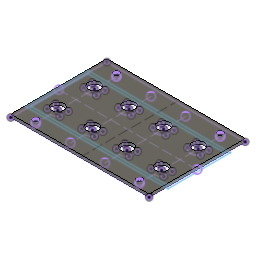
Compact ABR enclosure (Autodesk Fusion 360 archive; units mm, degrees)
design "ABR box faceplate"
Autodesk Fusion 360 part; units mm, degrees
sketch "Sketch1" plane through (0, 0, 0) normal (0, 0, 1) x (1, 0, 0)
  circle A0 centre (9, 34.525) radius 3.95
  circle A1 centre (9, 15.475) radius 3.95
  line L0 (9, 34.525) -> (9, 15.475) construction
  circle A2 centre (9, 45.975) radius 1.5
  circle A3 centre (9, 4.025) radius 1.5
  line L1 (-1.2896, 25) -> (19.2896, 25) construction
  line L2 (9, 45.975) -> (9, 4.025) construction
  line L3 (5.7, 40.3994) -> (5.7, 10.52)
  line L4 (5.7, 10.52) -> (12.3, 10.52) construction
  line L5 (12.3, 10.52) -> (12.3, 40.3994)
  line L6 (12.3, 40.3994) -> (5.7, 40.3994) construction
  line L7 (5.05, 34.525) -> (12.95, 34.525) construction
  circle A4 centre (27, 34.525) radius 3.95
  line L8 (23.7, 40.3994) -> (23.7, 10.52)
  line L9 (30.3, 10.52) -> (30.3, 40.3994)
  circle A5 centre (27, 15.475) radius 3.95
  circle A6 centre (27, 4.025) radius 1.5
  circle A7 centre (27, 45.975) radius 1.5
  circle A8 centre (45, 34.525) radius 3.95
  line L10 (41.7, 40.3994) -> (41.7, 10.52)
  line L11 (48.3, 10.52) -> (48.3, 40.3994)
  circle A9 centre (45, 15.475) radius 3.95
  circle A10 centre (45, 4.025) radius 1.5
  circle A11 centre (45, 45.975) radius 1.5
  line L12 (0, 50) -> (72, 50)
  line L13 (72, 50) -> (72, 0)
  line L14 (72, 0) -> (0, 0)
  line L15 (0, 0) -> (0, 50)
  line L16 (27, 45.975) -> (27, 4.025) construction
  line L17 (45, 45.975) -> (45, 4.025) construction
  circle A12 centre (63, 34.525) radius 3.95
  line L18 (59.7, 40.3994) -> (59.7, 10.52)
  line L19 (66.3, 10.52) -> (66.3, 40.3994)
  circle A13 centre (63, 15.475) radius 3.95
  circle A14 centre (63, 4.025) radius 1.5
  circle A15 centre (63, 45.975) radius 1.5
  line L20 (63, 45.975) -> (63, 4.025) construction
  line L21 (36, 50) -> (36, 0) construction
  line L22 (0, 25) -> (72, 25) construction
  line L23 (9, 15.475) -> (27, 15.475) construction
  line L24 (18, 15.475) -> (18, 27.912) construction
  point P0 (9, 5.525)
  point P1 (9, 11.525)
  point P2 (27, 34.525)
  point P3 (27, 15.475)
  point P4 (45, 34.525)
  point P5 (45, 15.475)
  point P6 (63, 34.525)
  point P7 (63, 15.475)
  point P8 (45, -15.475)
  point P9 (0, -50)
  point P10 (0, -25)
  point P11 (45, -45.975)
  point P12 (45, -34.525)
  point P13 (0, 50)
  dimension "d4" = 7.9
  dimension "d5" = 7.9
  dimension "d6" = 19.05
  dimension "d7" = 6
  dimension "d8" = 3
  dimension "d9" = 0.65
  dimension "d12" = 18
  dimension "d13" = 0
  dimension "d19" = 50
  dimension "d24" = 41.95
  dimension "d34" = 9
  dimension "d35" = 9
  dimension "d36" = 9
  constraint coincident A0.centre L0.start
  constraint coincident A1.centre L0.end
  constraint vertical L0
  constraint coincident L0 A2.centre
  constraint coincident L0 A3.centre
  constraint horizontal L1
  constraint midpoint L0 L1
  constraint symmetric A2 A3 L1
  constraint coincident A2.centre L2.start
  constraint coincident A3.centre L2.end
  constraint coincident A3 P0
  constraint coincident L2 P0
  constraint coincident L2 P1
  constraint coincident A1 P1
  constraint vertical L3
  constraint perpendicular L3 L4
  constraint perpendicular L4 L5
  constraint symmetric L2 L3 L5
  constraint horizontal L6
  constraint coincident A0 L7.start
  constraint coincident A0 L7.end
  constraint perpendicular L5 L7
  constraint coincident A0.centre L7
  constraint horizontal L12
  constraint vertical L13
  constraint horizontal L14
  constraint vertical L15
  constraint midpoint L12 L21.start
  constraint midpoint L14 L21.end
  constraint midpoint L15 L22.start
  constraint midpoint L13 L22.end
  constraint coincident L1 L22.start
  constraint coincident P3 A5.centre
  constraint midpoint L23 L24.start
  constraint perpendicular L1 L24
  constraint coincident L14.end L15.start
  measures "d4" diameter of A0
  measures "d5" diameter of A1
  measures "d6" distance of A0.centre A1.centre
  measures "d7" distance of P0 P1
  measures "d8" diameter of A3
  measures "d9" distance of L5 L7.end
  measures "d19" distance of P13 L14.end
  measures "d24" distance of A2.centre A3.centre
  measures "d34" distance of L0 L24
  measures "d35" distance of L2 L15
  measures "d36" distance of L13 L20
extrude "Extrude1" add sketch "Sketch1" along normal blind 1.5 contours A0 L5 | A0 A1 L3 L5 | A0 L3 | A1 L5 | A1 L3 | A4 L9 | A4 L8 L9 A5 | A4 L8 | L9 A5 | L8 A5 | A6 | A7 | A8 L11 | A8 L10 L11 A9 | A8 L10 | L11 A9 | L10 A9 | A10 | A11 | L12 L13 L14 L15 | A12 L19 | A12 L18 L19 A13 | A12 L18 | L19 A13 | L18 A13 makes body 1
sketch "Sketch2" plane through (0, 0, 0) normal (0, 0, -1) x (1, 0, 0)
  circle A0 centre (9, -4.025) radius 1.5
  circle A1 centre (63, -4.025) radius 1.5
  arc A2 (12.3, -13.3042) -> (5.7, -13.3042) centre (9, -15.475) ccw construction
  line L0 (12.3, -13.3042) -> (12.3, -17.6458) construction
  arc A3 (5.7, -17.6458) -> (12.3, -17.6458) centre (9, -15.475) ccw construction
  line L1 (5.7, -17.6458) -> (5.7, -13.3042) construction
  line L2 (30.3, -13.3042) -> (30.3, -17.6458) construction
  arc A4 (23.7, -17.6458) -> (30.3, -17.6458) centre (27, -15.475) ccw construction
  line L3 (23.7, -17.6458) -> (23.7, -13.3042) construction
  arc A5 (30.3, -13.3042) -> (23.7, -13.3042) centre (27, -15.475) ccw construction
  circle A6 centre (63, -45.975) radius 1.5
  line L4 (48.3, -13.3042) -> (48.3, -17.6458) construction
  arc A7 (41.7, -17.6458) -> (48.3, -17.6458) centre (45, -15.475) ccw construction
  line L5 (41.7, -17.6458) -> (41.7, -13.3042) construction
  arc A8 (48.3, -13.3042) -> (41.7, -13.3042) centre (45, -15.475) ccw construction
  circle A9 centre (9, -45.975) radius 1.5
  line L6 (66.3, -13.3042) -> (66.3, -17.6458) construction
  arc A10 (59.7, -17.6458) -> (66.3, -17.6458) centre (63, -15.475) ccw construction
  line L7 (59.7, -17.6458) -> (59.7, -13.3042) construction
  arc A11 (66.3, -13.3042) -> (59.7, -13.3042) centre (63, -15.475) ccw construction
  line L8 (72, 0) -> (0, 0)
  line L9 (0, 0) -> (0, -50)
  line L10 (0, -50) -> (72, -50)
  line L11 (72, -50) -> (72, 0)
  line L12 (0.4311, -10.2537) -> (71.5689, -10.2537)
  line L13 (71.5689, -10.2537) -> (71.5689, -39.7463)
  line L14 (71.5689, -39.7463) -> (0.4311, -39.7463)
  line L15 (0.4311, -39.7463) -> (0.4311, -10.2537)
  line L16 (0, -25) -> (72, -25) construction
  line L17 (27, -45.975) -> (27, -4.025) construction
  line L18 (45, -45.975) -> (45, -4.025) construction
  line L19 (63, -45.975) -> (63, -4.025) construction
  line L20 (9, -45.975) -> (9, -4.025) construction
  line L21 (36, 0) -> (36, -50) construction
  line L22 (73.0689, -8.7537) -> (73.0689, -41.2463)
  line L23 (73.0689, -41.2463) -> (-1.0689, -41.2463)
  line L24 (-1.0689, -41.2463) -> (-1.0689, -8.7537)
  line L25 (-1.0689, -8.7537) -> (73.0689, -8.7537)
  arc A12 (12.3, -32.3542) -> (5.7, -32.3542) centre (9, -34.525) ccw
  line L26 (12.3, -32.3542) -> (12.3, -36.6958)
  arc A13 (5.7, -36.6958) -> (12.3, -36.6958) centre (9, -34.525) ccw
  line L27 (5.7, -36.6958) -> (5.7, -32.3542)
  arc A14 (66.3, -32.3542) -> (59.7, -32.3542) centre (63, -34.525) ccw
  line L28 (66.3, -32.3542) -> (66.3, -36.6958)
  arc A15 (59.7, -36.6958) -> (66.3, -36.6958) centre (63, -34.525) ccw
  line L29 (59.7, -36.6958) -> (59.7, -32.3542)
  arc A16 (30.3, -32.3542) -> (23.7, -32.3542) centre (27, -34.525) ccw
  line L30 (30.3, -32.3542) -> (30.3, -36.6958)
  arc A17 (23.7, -36.6958) -> (30.3, -36.6958) centre (27, -34.525) ccw
  line L31 (23.7, -36.6958) -> (23.7, -32.3542)
  arc A18 (48.3, -32.3542) -> (41.7, -32.3542) centre (45, -34.525) ccw
  line L32 (48.3, -32.3542) -> (48.3, -36.6958)
  arc A19 (41.7, -36.6958) -> (48.3, -36.6958) centre (45, -34.525) ccw
  line L33 (41.7, -36.6958) -> (41.7, -32.3542)
  dimension "d18" = -1.5
  constraint horizontal L12
  constraint vertical L13
  constraint horizontal L14
  constraint vertical L15
  constraint midpoint L8 L21.start
  constraint midpoint L10 L21.end
  constraint symmetric L12 L14 L16
sketch "Sketch3" plane through (0, 0, 0) normal (0, 0, 1) x (1, 0, 0)
  line L0 (0, 50) -> (72, 50)
  line L1 (72, 50) -> (72, 0)
  line L2 (72, 0) -> (0, 0)
  line L3 (0, 0) -> (0, 50)
  circle A0 centre (9, 45.975) radius 1.5
  circle A1 centre (9, 4.025) radius 1.5
  circle A2 centre (9, 34.525) radius 3.15
  circle A3 centre (9, 15.475) radius 3.15
  circle A4 centre (27, 34.525) radius 3.15
  circle A5 centre (27, 45.975) radius 1.5
  circle A6 centre (27, 15.475) radius 3.15
  circle A7 centre (27, 4.025) radius 1.5
  circle A8 centre (45, 34.525) radius 3.15
  circle A9 centre (45, 45.975) radius 1.5
  circle A10 centre (45, 15.475) radius 3.15
  circle A11 centre (45, 4.025) radius 1.5
  circle A12 centre (63, 34.525) radius 3.15
  circle A13 centre (63, 45.975) radius 1.5
  circle A14 centre (63, 15.475) radius 3.15
  circle A15 centre (63, 4.025) radius 1.5
  point P0 (0, 50)
  point P1 (72, 0)
  point P2 (9, 45.975)
  point P3 (9, 4.025)
  point P4 (9, 34.525)
  point P5 (9, 15.475)
  point P6 (27, 15.475)
  point P7 (27, 4.025)
  point P8 (45, 15.475)
  point P9 (45, 4.025)
  point P10 (63, 15.475)
  point P11 (63, 4.025)
  dimension "d25" = 6.3
  dimension "d26" = 6.3
  dimension "d29" = 18
  dimension "d30" = 0
  constraint horizontal L0
  constraint vertical L1
  constraint horizontal L2
  constraint vertical L3
  constraint coincident P1 L1.end
  constraint coincident P0 L0.start
  constraint coincident P4 A2.centre
  constraint coincident P5 A3.centre
  measures "d25" diameter of A2
  measures "d26" diameter of A3
extrude "Extrude3" add sketch "Sketch3" along normal blind 1.5 separate body contours L0 L1 L2 L3 | A5 | A7 | A9 | A11 makes body 2
fillet "Fillet1" radius 1 4 edges at (72, 0, 0.75) (0, 0, 0.75) (72, 50, 0.75) (0, 50, 0.75) on bodies 2
hidden bodies 1
equation "banana_d = 7.9 mm"
equation "ctr_to_ctr = 0.75 in"
equation "flat_inset = 0.65 mm"
equation "d4 = banana_d"
equation "d5 = banana_d"
equation "d6 = ctr_to_ctr"
equation "d7 = 5 mm + 1 mm"
equation "d9 = flat_inset"
equation "x_spacing = 18 mm"
equation "d26 = d25"
equation "d29 = x_spacing"
equation "d36 = d35"
named bodies: "Bananas_faceplate", "bana solder lug faceplate"
